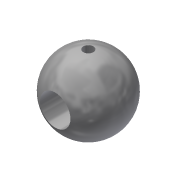
# Autodesk Inventor part: Handle_Ball
Saved by Autodesk Inventor 2022 Beta2 (Build 260130000, 130) ContinuousBuild 0
## iProperties
Created: 2006-01-18
Part Number: Handle_Ball
Document SubType Name: Modeling
Designer: PMiller
Material: Steel, Mild
Density: 7.86 g/cm^3
Appearance: Steel
Author: PMiller
Autodesk Inventor part; units mm, degrees
ref_plane "YZ Plane" through (0, 0, 0) normal (1, 0, 0) x (0, 1, 0)
ref_plane "XZ Plane" through (0, 0, 0) normal (0, 1, 0) x (-1, 0, 0)
sketch "Sketch1" plane through (0, 0, 0) normal (0, 0, 1) x (1, 0, 0)
  line L0 (0, 9.525) -> (0, -9.525)
  arc A0 (0, -9.525) -> (0, 9.525) centre (0, 0) ccw
  dimension "d0" = 9.525
  constraints: 2 coincident, 2 end point, 2 point on circle, 1 centre point, 1 midpoint, 1 vertical
  measures "d0" radius of A0
revolve "Revolution1" add sketch "Sketch1" angle 360 about axis through (0, 9.525, 0) along (0, -1, 0)
ref_plane "Work Plane1" through (0, 0, 9.525) normal (0, 0, 1) x (1, 0, 0)
sketch "Sketch2" plane through (0, 0, 9.525) normal (0, 0, 1) x (1, 0, 0)
  circle A0 centre (0, 0) radius 3.9751
  dimension "d2" = 7.9502
  constraints: 1 centre point, 1 coincident
  measures "d2" diameter of A0
extrude "Extrusion1" cut sketch "Sketch2" against normal blind 12.7
sketch "Sketch3" plane through (0, 0, 0) normal (0, 1, 0) x (-1, 0, 0)
  circle A0 centre (0, 0) radius 1.3208
  dimension "d5" = 2.6416
  constraints: 1 centre point, 1 coincident
  measures "d5" diameter of A0
extrude "Extrusion2" cut sketch "Sketch3" along normal through all both and the other way through all
body "Solid1"
